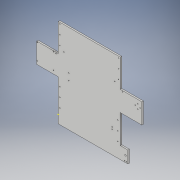
# Autodesk Inventor part: Gen2PlatePart
Saved by Autodesk Inventor 2017 (Build 210142000, 142)
## iProperties
Created: 2017-12-06
Part Number: Gen2PlatePart
Material: Generic
Document SubType Name: Modeling
Designer: User
Density: 1 g/cm^3
Appearance: Default
Author: User
Autodesk Inventor part; units mm, degrees
ref_plane "YZ Plane" through (0, 0, 0) normal (1, 0, 0) x (0, 1, 0)
ref_plane "XZ Plane" through (0, 0, 0) normal (0, 1, 0) x (-1, 0, 0)
ref_plane "XY Plane" through (0, 0, 0) normal (0, 0, 1) x (1, 0, 0)
sketch "Sketch1" plane through (0, 0, 0) normal (0, 0, 1) x (1, 0, 0)
  line L0 (0, 0) -> (254, 0)
  line L1 (254, 0) -> (254, 330.2)
  line L2 (254, 330.2) -> (0, 330.2)
  line L3 (0, 330.2) -> (0, 0)
  dimension "d0" = 254
  dimension "d1" = 330.2
  constraints: 8 end point, 2 parallel, 1 horizontal, 1 perpendicular
  measures "d0" distance of L2.end L1.end
  measures "d1" distance of L1.end L0.end
extrude "Extrusion1" add sketch "Sketch1" along normal blind 6.35
sketch "Sketch2" plane through (0, 0, 6.35) normal (0, 0, 1) x (1, 0, 0)
  point P0 (0, 0)
sketch "Sketch3" plane through (0, 0, 0) normal (-1, 0, 0) x (0, 0, 1)
  line L0 (0, 0) -> (0, 330.2) projected
  line L1 (0, 330.2) -> (-38.1, 330.2)
  line L2 (-38.1, 330.2) -> (38.1, 330.2)
  line L3 (38.1, 330.2) -> (38.1, 266.7)
  line L4 (38.1, 266.7) -> (-38.1, 266.7)
  line L5 (-38.1, 266.7) -> (-38.1, 330.2)
  line L6 (-38.1, 0) -> (38.1, 0)
  line L7 (38.1, 0) -> (38.1, 63.5)
  line L8 (38.1, 63.5) -> (-38.1, 63.5)
  line L9 (-38.1, 63.5) -> (-38.1, 0)
  dimension "d4" = 38.1
  dimension "d5" = 76.2
  dimension "d6" = 63.5
  dimension "d9" = 63.5
  constraints: 18 end point, 4 parallel, 3 horizontal, 2 perpendicular
  measures "d4" distance of L0.end L1.end
  measures "d5" distance of L3.end L4.end
  measures "d6" distance of L2.end L3.end
  measures "d9" distance of L7.end L6.end
extrude "Extrusion2" add sketch "Sketch3" against normal blind 6.35
sketch "Sketch4" plane through (6.35, 0, 0) normal (0, -1, 0) x (1, 0, 0)
  line L0 (0, -38.1) -> (0, 0) projected
  line L1 (247.65, 6.35) -> (0, 6.35) projected
  line L2 (0, 0) -> (38.1, 0)
  line L3 (38.1, 0) -> (38.1, 6.35)
  line L4 (38.1, 6.35) -> (0, 6.35)
  line L5 (0, 6.35) -> (0, 0)
  point P0 (-6.35, 0)
  dimension "d10" = 38.1
  constraints: 8 end point, 2 parallel, 1 horizontal, 1 perpendicular, 1 point on line
  measures "d10" distance of L4.end L3.end
extrude "Extrusion3" cut sketch "Sketch4" against normal blind 38.1
sketch "Sketch5" plane through (6.35, 330.2, 0) normal (0, 1, 0) x (1, 0, 0)
  line L0 (0, 0) -> (-6.35, 0) projected
  line L1 (0, -6.35) -> (38.1, -6.35) projected
  line L2 (0, 0) -> (38.1, 0)
  line L3 (38.1, 0) -> (38.1, -6.35)
  line L4 (38.1, -6.35) -> (0, -6.35)
  line L5 (0, -6.35) -> (0, 0)
  constraints: 8 end point, 2 parallel, 1 horizontal, 1 perpendicular
extrude "Extrusion4" cut sketch "Sketch5" against normal blind 38.1
sketch "Sketch6" plane through (254, 0, 0) normal (1, 0, 0) x (0, 0, -1)
  line L0 (38.1, 0) -> (-38.1, 0) projected
  line L1 (38.1, 63.5) -> (0, 63.5) projected
  line L2 (-38.1, 0) -> (38.1, 0)
  line L3 (38.1, 0) -> (38.1, 63.5)
  line L4 (38.1, 63.5) -> (-38.1, 63.5)
  line L5 (-38.1, 63.5) -> (-38.1, 0)
  line L6 (-38.1, 266.7) -> (-6.35, 266.7) projected
  line L7 (38.1, 330.2) -> (-38.1, 330.2) projected
  line L8 (-38.1, 266.7) -> (38.1, 266.7)
  line L9 (38.1, 266.7) -> (38.1, 330.2)
  line L10 (38.1, 330.2) -> (-38.1, 330.2)
  line L11 (-38.1, 330.2) -> (-38.1, 266.7)
  point P0 (0, 0)
  constraints: 16 end point, 4 parallel, 2 horizontal, 2 perpendicular
extrude "Extrusion5" add sketch "Sketch6" against normal blind 6.35
sketch "Sketch7" plane through (44.45, 330.2, 6.35) normal (0, 1, 0) x (1, 0, 0)
  line L0 (0, 0) -> (203.2, 0) projected
  line L1 (0, 6.35) -> (203.2, 6.35) projected
  line L2 (203.2, 0) -> (165.1, 0)
  line L3 (165.1, 0) -> (165.1, 6.35)
  line L4 (165.1, 6.35) -> (203.2, 6.35)
  line L5 (203.2, 6.35) -> (203.2, 0)
  point P0 (-44.45, 6.35)
  dimension "d17" = 38.1
  constraints: 8 end point, 2 parallel, 1 horizontal, 1 perpendicular, 1 point on line
  measures "d17" distance of L3.end L4.end
extrude "Extrusion6" cut sketch "Sketch7" against normal blind 38.1
sketch "Sketch8" plane through (44.45, 0, 0) normal (0, -1, 0) x (1, 0, 0)
  line L0 (209.55, 0) -> (203.2, 0) projected
  line L1 (0, 6.35) -> (203.2, 6.35) projected
  line L2 (203.2, 0) -> (165.1, 0)
  line L3 (165.1, 0) -> (165.1, 6.35)
  line L4 (165.1, 6.35) -> (203.2, 6.35)
  line L5 (203.2, 6.35) -> (203.2, 0)
  point P0 (-44.45, 0)
  dimension "d20" = 38.1
  constraints: 8 end point, 2 parallel, 1 horizontal, 1 perpendicular, 1 point on line
  measures "d20" distance of L3.end L4.end
extrude "Extrusion7" cut sketch "Sketch8" against normal blind 38.1
sketch "Sketch9" plane through (6.35, 0, 0) normal (1, 0, 0) x (0, 0, -1)
  line L0 (38.1, 0) -> (-38.1, 0) projected
  line L1 (-19.0903, 0) -> (-19.0903, 17.1196)
  line L2 (-19.0903, 0) -> (-1.9707, 0) construction
  line L3 (-38.1, 63.5) -> (-38.1, 0) projected
  line L4 (-38.1, 17.1196) -> (-20.955, 17.1196)
  line L5 (-38.1, 17.1196) -> (-20.955, 17.1196) construction
  circle A0 centre (-20.955, 17.1196) radius 3.4925
  point P0 (0, 0)
  dimension "d23" = 17.1196
  dimension "d24" = 90
  dimension "d25" = 17.145
  dimension "d26" = 0
  dimension "d27" = 6.985
  constraints: 8 end point, 2 equal length, 2 horizontal, 2 perpendicular, 2 point on line, 1 centre point, 1 coincident
  measures "d23" distance of L1.start L1.end
  measures "d24" angle of L2 L1
  measures "d25" distance of L4.start L4.end
  measures "d26" distance between parallel lines of L4 L5
  measures "d27" diameter of A0
extrude "Extrusion8" cut sketch "Sketch9" against normal blind 38.1 contours A0
sketch "Sketch10" plane through (6.35, 0, 0) normal (1, 0, 0) x (0, 0, -1)
  circle A0 centre (-20.955, 17.1196) radius 3.4925 projected
  circle A1 centre (-20.955, 17.1196) radius 8
  circle A2 centre (-20.955, 9.1196) radius 1.5875
  circle A3 centre (-14.0268, 13.1196) radius 1.5875
  circle A4 centre (-20.955, 17.1196) radius 8
  circle A5 centre (-14.0268, 21.1196) radius 1.5875
  circle A6 centre (-20.955, 17.1196) radius 8
  circle A7 centre (-20.955, 25.1196) radius 1.5875
  circle A8 centre (-20.955, 17.1196) radius 8
  circle A9 centre (-27.8832, 21.1196) radius 1.5875
  circle A10 centre (-20.955, 17.1196) radius 8
  circle A11 centre (-27.8832, 13.1196) radius 1.5875
  circle A12 centre (-20.955, 17.1196) radius 8
  point P0 (0, 0)
  point P1 (-28.955, 17.1196)
  point P2 (-24.955, 10.1914)
  point P3 (-16.955, 10.1914)
  point P4 (-12.955, 17.1196)
  point P5 (-16.955, 24.0478)
  point P6 (-24.955, 24.0478)
  dimension "d33" = 3.175
  dimension "d36" = 360
  constraints: 12 centre point, 12 point on circle, 9 coincident, 35 other
  measures "d33" diameter of A2
extrude "Extrusion9" cut sketch "Sketch10" against normal blind 38.1 contours A5 A1 | A1 A5 | A3 A1 | A1 A3 | A7 A1 | A1 A7 | A2 A1 | A1 A2 | A9 A1 | A1 A9 | A11 A1 | A1 A11
sketch "Sketch11" plane through (247.65, 0, 0) normal (-1, 0, 0) x (0, 0, 1)
  line L0 (38.1, 0) -> (38.1, 63.5) projected
  line L1 (38.1, 17.1196) -> (70.485, 17.1196) construction
  circle A0 centre (20.955, 17.1196) radius 3.4925
  circle A1 centre (20.955, 17.1196) radius 8.001
  line L2 (20.955, 17.1196) -> (31.4906, 17.1196)
  circle A2 centre (28.956, 17.1196) radius 1.5875
  circle A3 centre (24.9555, 24.0487) radius 1.5875
  circle A4 centre (20.955, 17.1196) radius 8.001
  circle A5 centre (16.9545, 24.0487) radius 1.5875
  circle A6 centre (20.955, 17.1196) radius 8.001
  circle A7 centre (12.954, 17.1196) radius 1.5875
  circle A8 centre (20.955, 17.1196) radius 8.001
  circle A9 centre (16.9545, 10.1905) radius 1.5875
  circle A10 centre (20.955, 17.1196) radius 8.001
  circle A11 centre (24.9555, 10.1905) radius 1.5875
  circle A12 centre (20.955, 17.1196) radius 8.001
  point P0 (0, 0)
  point P1 (20.955, 9.1186)
  point P2 (27.8841, 13.1191)
  point P3 (27.8841, 21.1201)
  point P4 (20.955, 25.1206)
  point P5 (14.0259, 21.1201)
  point P6 (14.0259, 13.1191)
  dimension "d44" = 16.002
  dimension "d41" = 17.145
  dimension "d43" = 6.985
  dimension "d81" = 3.175
  dimension "d84" = 360
  constraints: 7 centre point, 4 end point, 3 coincident, 2 point on line, 2 vertical alignment, 1 horizontal, 47 other
  measures "d41" distance of L1.start point (20.955, 17.12)
  measures "d43" diameter of A0
  measures "d81" diameter of A2
extrude "Extrusion10" cut sketch "Sketch11" against normal blind 25.4 contours A0 | L2 A2 A1 | L2 A2 A1 | A1 A2 L2 | A1 A2 L2 | A3 A1 | A1 A3 | A11 A1 | A1 A11 | A5 A1 | A1 A5 | A9 A1 | A1 A9 | A7 A1 | A1 A7
sketch "Sketch12" plane through (254, 63.5, 0) normal (1, 0, 0) x (0, 0, -1)
  line L0 (-38.1, 266.7) -> (-38.1, 203.2) projected
  line L1 (-38.1, 234.95) -> (-20.955, 234.95)
  line L2 (0, 228.6) -> (0, 266.7) projected
  line L3 (38.1, 266.7) -> (-38.1, 266.7) projected
  line L4 (-20.955, 266.7) -> (-20.955, 249.5804)
  line L5 (-20.955, 266.7) -> (-3.8354, 266.7) construction
  circle A0 centre (-20.955, 249.5804) radius 3.4925
  circle A1 centre (-20.955, 249.5804) radius 8.001
  line L6 (-20.955, 234.95) -> (-20.955, 230.7922)
  line L7 (-20.955, 249.5804) -> (-30.6683, 249.5804)
  line L8 (-6.35, 266.7) -> (-6.35, 228.6) projected
  circle A2 centre (-20.955, 257.5814) radius 1.5875
  circle A3 centre (-27.8841, 253.5809) radius 1.5875
  circle A4 centre (-20.955, 249.5804) radius 8.001
  circle A5 centre (-27.8841, 245.5799) radius 1.5875
  circle A6 centre (-20.955, 249.5804) radius 8.001
  circle A7 centre (-20.955, 241.5794) radius 1.5875
  circle A8 centre (-20.955, 249.5804) radius 8.001
  circle A9 centre (-14.0259, 245.5799) radius 1.5875
  circle A10 centre (-20.955, 249.5804) radius 8.001
  circle A11 centre (-14.0259, 253.5809) radius 1.5875
  circle A12 centre (-20.955, 249.5804) radius 8.001
  point P0 (0, -63.5)
  dimension "d56" = 16.002
  dimension "d52" = 17.145
  dimension "d53" = 17.1196
  dimension "d54" = 90
  dimension "d55" = 6.985
  dimension "d80" = 0
  dimension "d104" = 3.175
  dimension "d107" = 360
  constraints: 10 end point, 8 coincident, 7 centre point, 4 perpendicular, 2 point on line, 2 vertical alignment, 1 horizontal, 1 midpoint, 1 vertical, 47 other
  measures "d52" distance of L1.start L1.end
  measures "d53" distance of L4.start L4.end
  measures "d54" angle of L4 L5
  measures "d55" diameter of A0
  measures "d80" distance from line of L4.end L6
  measures "d104" diameter of A2
extrude "Extrusion11" cut sketch "Sketch12" against normal blind 25.4 contours A2 A1 L4 | L4 A1 A2 | A1 A2 L4 | L4 A2 A1 | A3 A1 | A1 A3 | A0 L7 L4 | L4 L7 A0 | A11 A1 | A1 A11 | A5 A1 | A1 A5 | A9 A1 | A1 A9 | A7 A1 | A1 A7
sketch "Sketch13" plane through (0, 63.5, 0) normal (-1, 0, 0) x (0, 0, 1)
  line L0 (-38.1, 266.7) -> (38.1, 266.7) projected
  line L1 (23.9735, 266.7) -> (41.0931, 266.7) construction
  line L2 (38.1, 249.5804) -> (20.955, 249.5804)
  line L3 (38.1, 249.5804) -> (55.245, 249.5804) construction
  circle A0 centre (20.955, -46.3804) radius 3.4925 projected
  line L4 (38.1, -63.5) -> (38.1, 0) projected
  circle A1 centre (20.955, 249.5804) radius 3.4925
  circle A2 centre (20.955, 249.5804) radius 8.001
  circle A3 centre (28.956, 249.5804) radius 1.5875
  circle A4 centre (24.9555, 256.5095) radius 1.5875
  circle A5 centre (20.955, 249.5804) radius 8.001
  circle A6 centre (16.9545, 256.5095) radius 1.5875
  circle A7 centre (20.955, 249.5804) radius 8.001
  circle A8 centre (12.954, 249.5804) radius 1.5875
  circle A9 centre (20.955, 249.5804) radius 8.001
  circle A10 centre (16.9545, 242.6513) radius 1.5875
  circle A11 centre (20.955, 249.5804) radius 8.001
  circle A12 centre (24.9555, 242.6513) radius 1.5875
  circle A13 centre (20.955, 249.5804) radius 8.001
  line L5 (38.1, 203.2) -> (6.35, 203.2) projected
  point P0 (0, -63.5)
  point P1 (20.9804, 257.5814)
  point P2 (14.0387, 253.6029)
  point P3 (14.0133, 245.6019)
  point P4 (20.9296, 241.5794)
  point P5 (27.8713, 245.5579)
  point P6 (27.8967, 253.5589)
  dimension "d67" = 17.145
  dimension "d68" = 180
  dimension "d69" = 17.145
  dimension "d70" = 6.985
  dimension "d71" = 6.985
  dimension "d72" = 16.002
  dimension "d92" = 3.175
  dimension "d95" = 360
  dimension "d134" = 46.3804
  constraints: 13 centre point, 12 point on circle, 6 end point, 3 horizontal, 2 coincident, 2 point on line, 1 collinear, 31 other
  measures "d67" distance of L2.start L2.end
  measures "d68" angle of L2 L3
  measures "d69" distance from line of A0.centre L4
  measures "d70" diameter of A0
  measures "d71" diameter of A1
  measures "d72" diameter of A2
  measures "d92" diameter of A3
  measures "d134" distance from line of L5 L2.end
extrude "Extrusion12" cut sketch "Sketch13" against normal blind 25.4 contours A3 A2 L2 | L2 A2 A3 | A2 A3 L2 | L2 A3 A2 | A4 A2 | A2 A4 | A12 A2 | A2 A12 | A6 A2 | A2 A6 | A10 A2 | A2 A10 | A8 A2 | A2 A8 | A1
sketch "Sketch14" plane through (254, 63.5, 0) normal (1, 0, 0) x (0, 0, -1)
  line L0 (0, -63.5) -> (0, 50.8)
  line L1 (0, 203.2) -> (0, 0) projected
  line L2 (38.1, 266.7) -> (-38.1, 266.7) projected
  line L3 (0, 266.7) -> (0, 165.1)
  line L4 (-6.35, 203.2) -> (-6.35, 0) projected
  line L5 (0, 50.8) -> (-6.35, 50.8)
  line L6 (-6.35, 241.3) -> (0, 241.3)
  line L7 (0, 266.7) -> (-6.35, 266.7) projected
  line L8 (0, 266.7) -> (0, 152.4)
  line L9 (0, 0) -> (0, 203.2) projected
  line L10 (-6.35, 0) -> (-6.35, 203.2) projected
  line L11 (0, 50.8) -> (-6.35, 50.8)
  line L12 (-6.35, 152.4) -> (0, 152.4)
  line L13 (0, 152.4) -> (0, 69.85)
  line L14 (0, 69.85) -> (-6.35, 69.85)
  line L15 (-6.35, 69.85) -> (-6.35, 152.4)
  dimension "d109" = 114.3
  dimension "d137" = 114.3
  dimension "d305" = 82.55
  constraints: 20 end point, 5 point on line, 2 horizontal, 2 parallel, 1 collinear, 1 midpoint, 1 perpendicular
  measures "d109" distance of L0.start L0.end
  measures "d137" distance of L3.start L8.end
  measures "d305" distance of L12.end L13.end
sketch "Sketch15" plane through (0, 63.5, 0) normal (-1, 0, 0) x (0, 0, 1)
  line L0 (0, -63.5) -> (0, 38.1)
  line L1 (0, 0) -> (0, -25.4) projected
  line L2 (-38.1, 266.7) -> (38.1, 266.7) projected
  line L3 (0, 266.7) -> (0, 165.1)
  line L4 (0, 266.7) -> (0, 228.6) projected
  line L5 (0, 165.1) -> (6.35, 165.1)
  line L6 (6.35, 38.1) -> (0, 38.1)
  line L7 (0, 165.1) -> (0, 69.85)
  line L8 (0, 69.85) -> (6.35, 69.85)
  line L9 (6.35, 165.1) -> (6.35, 69.85)
  line L10 (6.35, 203.2) -> (6.35, 0) projected
  dimension "d113" = 101.6
  dimension "d114" = 101.6
  dimension "d306" = 95.25
  constraints: 14 end point, 3 collinear, 1 horizontal, 1 midpoint, 1 parallel
  measures "d113" distance of L0.start L0.end
  measures "d114" distance of L3.start L3.end
  measures "d306" distance of L3.end L7.end
extrude "Extrusion14" add sketch "Sketch15" along normal blind 88.9
thicken "Thicken1" operation add thickness 22.225 both sides no extend neighbours yes toward (0, 0, 1) faces at (251.8833, 287.8667, -38.1)
thicken "Thicken2" operation add thickness 22.225 both sides no extend neighbours yes toward (0, 0, 1) faces at (2.1167, 287.8667, -38.1)
thicken "Thicken3" operation add thickness 22.225 both sides no extend neighbours yes toward (0, 0, 1) faces at (2.1167, 42.3333, -38.1)
thicken "Thicken4" operation add thickness 22.225 both sides no extend neighbours yes toward (0, 0, 1) faces at (251.8833, 21.1667, -38.1)
extrude "Extrusion15" add sketch "Sketch14" along normal blind 88.9 contours L1 L14 L4 L12
thicken "Thicken10" operation add thickness 12.7 both sides no extend neighbours yes toward (0, -1, 0) faces at (-29.6333, 228.6, 4.2333)
thicken "Thicken12" operation add thickness 15.875 both sides no extend neighbours yes toward (0, 0, 1) faces at (249.7667, 309.0333, -15.875)
thicken "Thicken13" operation add thickness 15.875 both sides no extend neighbours yes toward (0, 0, 1) faces at (4.2333, 287.8667, -15.875)
thicken "Thicken14" operation add thickness 15.875 both sides no extend neighbours yes toward (0, 0, 1) faces at (251.8833, 21.1667, -15.875)
thicken "Thicken15" operation add thickness 15.875 both sides no extend neighbours yes toward (0, 0, 1) faces at (2.1167, 42.3333, -15.875)
thicken "Thicken16" operation add thickness 38.1 both sides no extend neighbours yes toward (-1, 0, 0) faces at (44.45, 25.4, 2.1167)
thicken "Thicken17" operation add thickness 38.1 both sides no extend neighbours yes toward (1, 0, 0) faces at (209.55, 25.4, 2.1167)
thicken "Thicken18" operation add thickness 38.1 both sides no extend neighbours yes toward (1, 0, 0) faces at (209.55, 317.5, 2.1167)
thicken "Thicken19" operation add thickness 38.1 both sides no extend neighbours yes toward (-1, 0, 0) faces at (44.45, 317.5, 2.1167)
thicken "Thicken20" operation add thickness 34.925 both sides no extend neighbours yes toward (0, -1, 0) faces at (86.7833, 0, 2.1167)
thicken "Thicken21" operation add thickness 12.7 both sides no extend neighbours yes toward (0, -1, 0) faces at (167.2167, -34.925, 2.1167)
thicken "Thicken22" operation add thickness 31.75 both sides no extend neighbours yes toward (0, 0, -1) faces at (2.1167, 309.0333, 38.1)
thicken "Thicken23" operation add thickness 31.75 both sides no extend neighbours yes toward (0, 0, -1) faces at (249.7667, 309.0333, 38.1)
thicken "Thicken24" operation add thickness 31.75 both sides no extend neighbours yes toward (0, 0, -1) faces at (4.2333, 26.4583, 38.1)
thicken "Thicken25" operation add thickness 31.75 both sides no extend neighbours yes toward (0, 0, -1) faces at (249.7667, -10.5833, 38.1)
sketch "Sketch20" plane through (0, 330.2, 6.35) normal (0, 0, 1) x (1, 0, 0)
  line L0 (0, -114.3) -> (0, 0) projected
  line L1 (0, 0) -> (12.7, 0)
  line L2 (12.7, 0) -> (12.7, -88.9)
  line L3 (12.7, -88.9) -> (0, -88.9)
  line L4 (0, -88.9) -> (0, 0)
  line L5 (254, -114.3) -> (254, 0) projected
  line L6 (254, 0) -> (241.3, 0)
  line L7 (241.3, 0) -> (241.3, -88.9)
  line L8 (241.3, -88.9) -> (254, -88.9)
  line L9 (254, -88.9) -> (254, 0)
  line L10 (254, -377.825) -> (254, 0) projected
  line L11 (254, -222.25) -> (233.7253, -222.25)
  line L12 (233.7253, -222.25) -> (233.7253, -311.15)
  line L13 (233.7253, -311.15) -> (254, -311.15)
  line L14 (254, -311.15) -> (254, -222.25)
  line L15 (0, -196.85) -> (0, -377.825) projected
  line L16 (0, -222.25) -> (12.7, -222.25)
  line L17 (12.7, -222.25) -> (12.7, -311.15)
  line L18 (12.7, -311.15) -> (0, -311.15)
  line L19 (0, -311.15) -> (0, -222.25)
  line L20 (6.35, -311.15) -> (6.35, -304.8)
  line L21 (0, -266.7) -> (12.7, -266.7)
  line L22 (6.35, -222.25) -> (6.35, -228.6)
  line L23 (233.7253, -266.7) -> (254, -266.7)
  line L24 (243.8627, -311.15) -> (243.8627, -304.8)
  line L25 (243.8627, -222.25) -> (243.8627, -228.6)
  line L26 (247.65, 0) -> (247.65, -6.35)
  line L27 (241.3, -44.45) -> (254, -44.45)
  line L28 (247.65, -88.9) -> (247.65, -82.55)
  line L29 (6.35, 0) -> (6.35, -6.35)
  line L30 (0, -44.45) -> (12.7, -44.45)
  line L31 (6.35, -88.9) -> (6.35, -82.55)
  line L32 (254, -215.9) -> (342.9, -215.9) projected
  line L33 (243.8627, -228.6) -> (6.35, -228.6)
  point P0 (0, -330.2)
  point P1 (0, -228.6)
  point P2 (6.35, -266.7)
  point P3 (243.8627, -266.7)
  point P4 (247.65, -44.45)
  point P5 (6.35, -44.45)
  dimension "d200" = 12.7
  dimension "d201" = 88.9
  dimension "d202" = 12.7
  dimension "d203" = 88.9
  dimension "d204" = 88.9
  dimension "d208" = 6.35
  dimension "d209" = 6.35
  dimension "d210" = 6.35
  dimension "d211" = 6.35
  dimension "d212" = 6.35
  dimension "d213" = 6.35
  dimension "d214" = 0
  dimension "d216" = 6.35
  dimension "d217" = 0
  dimension "d311" = 38.1
  dimension "d312" = 38.1
  dimension "d313" = 6.35
  dimension "d314" = 6.35
  dimension "d315" = 38.1
  dimension "d316" = 38.1
  dimension "d317" = 38.1
  dimension "d318" = 0
  constraints: 58 end point, 20 midpoint, 8 coincident, 8 parallel, 8 vertical, 5 horizontal, 4 perpendicular
  measures "d200" distance of L2.end L3.end
  measures "d201" distance of L1.end L2.end
  measures "d202" distance of L8.end L7.end
  measures "d203" distance of L7.end L6.end
  measures "d204" distance of L12.end L11.end
  measures "d208" distance of L24.start L24.end
  measures "d209" distance of L25.start L25.end
  measures "d210" distance of L26.start L26.end
  measures "d211" distance of L28.start L28.end
  measures "d212" distance of L29.start L29.end
  measures "d213" distance of L31.start L31.end
  measures "d214" distance between parallel lines of L15 L19
  measures "d216" distance between parallel lines of L32 L11
  measures "d217" distance between parallel lines of L10 L14
  measures "d311" distance of point (6.35, -266.7) point (6.35, -228.6)
  measures "d312" distance of point (6.35, -266.7) point (6.35, -304.8)
  measures "d313" distance of point (6.35, -228.6) L22.start
  measures "d314" distance of L20.start point (6.35, -304.8)
  measures "d315" distance of L33.start point (243.863, -266.7)
  measures "d316" distance of point (243.863, -304.8) point (243.863, -266.7)
  measures "d317" distance of point (6.35, -6.35) point (6.35, -44.45)
  measures "d318" distance of point (6.35, -228.6) L33.end
hole "Hole3" at (6.35, 323.85, 6.35) at (6.35, 285.75, 6.35) at (6.35, 247.65, 6.35) at (6.35, 101.6, 6.35) at (6.35, 63.5, 6.35) at (6.35, 25.4, 6.35) at (247.65, 285.75, 6.35) at (247.65, 323.85, 6.35) at (247.65, 247.65, 6.35) at (243.8627, 101.6, 6.35) at (243.8627, 63.5, 6.35) at (243.8627, 25.4, 6.35) direction (0, 0, -1) diameter 3.302 depth 25.4 tip angle 118
sketch "Sketch22" plane through (0, 330.2, 6.35) normal (0, 0, 1) x (1, 0, 0)
  line L0 (254, -114.3) -> (342.9, -114.3) projected
  line L1 (342.9, -114.3) -> (342.9, -215.9) projected
  circle A0 centre (335.915, -139.7) radius 1.778
  circle A1 centre (316.357, -139.7) radius 1.778
  circle A2 centre (325.882, -130.175) radius 1.778
  circle A3 centre (325.882, -149.225) radius 1.778
  point P0 (0, -330.2)
  dimension "d236" = 25.4
  dimension "d237" = 6.985
  dimension "d238" = 3.556
  dimension "d239" = 26.543
  dimension "d240" = 3.556
  dimension "d241" = 9.525
  dimension "d242" = 9.525
  dimension "d243" = 3.556
  dimension "d244" = 9.525
  dimension "d245" = 9.525
  dimension "d246" = 3.556
  constraints: 4 centre point, 4 coincident
  measures "d236" distance from line of L0 point (335.915, -139.7)
  measures "d237" distance from line of point (335.915, -139.7) L1
  measures "d238" diameter of A0
  measures "d239" distance from line of L1 point (316.357, -139.7)
  measures "d240" diameter of A1
  measures "d241" horizontal distance of point (325.882, -130.175) point (316.357, -139.7)
  measures "d242" horizontal distance of point (316.357, -139.7) point (325.882, -130.175)
  measures "d243" diameter of A2
  measures "d244" horizontal distance of point (325.882, -149.225) A1.centre
  measures "d245" horizontal distance of A1.centre point (325.882, -149.225)
  measures "d246" diameter of A3
extrude "Extrusion17" cut sketch "Sketch22" against normal blind 25.4
sketch "Sketch23" plane through (0, 330.2, 6.35) normal (0, 0, 1) x (1, 0, 0)
  circle A0 centre (325.882, -130.175) radius 1.778 projected
  circle A1 centre (335.915, -139.7) radius 1.778 projected
  circle A2 centre (316.357, -139.7) radius 1.778 projected
  circle A3 centre (325.882, -149.225) radius 1.778 projected
  circle A4 centre (243.8627, -266.7) radius 1.651 projected
  circle A5 centre (247.65, -82.55) radius 1.651 projected
  circle A6 centre (247.65, -44.45) radius 1.651 projected
  circle A7 centre (6.35, -266.7) radius 1.651 projected
  circle A8 centre (6.35, -82.55) radius 1.651 projected
  circle A9 centre (6.35, -6.35) radius 1.651 projected
  circle A10 centre (6.35, -44.45) radius 1.651 projected
  circle A11 centre (6.35, -228.6) radius 1.651 projected
  circle A12 centre (6.35, -304.8) radius 1.651 projected
  circle A13 centre (247.65, -6.35) radius 1.651 projected
  circle A14 centre (243.8627, -228.6) radius 1.651 projected
  circle A15 centre (243.8627, -304.8) radius 1.651 projected
  line L0 (254, 0) -> (254, -114.3) projected
  line L1 (254, -114.3) -> (342.9, -114.3) projected
  line L2 (0, 0) -> (254, 0) projected
  line L3 (0, 0) -> (0, -114.3) projected
  line L4 (0, -114.3) -> (-88.9, -114.3) projected
  line L5 (254, -377.825) -> (0, -377.825) projected
  line L6 (254, -196.85) -> (342.9, -196.85) projected
  line L7 (342.9, -114.3) -> (342.9, -196.85) projected
  line L8 (-88.9, -196.85) -> (-88.9, -114.3) projected
  line L9 (0, -196.85) -> (-88.9, -196.85) projected
  line L10 (0, -377.825) -> (0, -196.85) projected
  line L11 (254, -377.825) -> (254, -196.85) projected
  point P0 (0, -330.2)
  point P1 (263.1059, -119.0625)
  point P2 (231.3559, -97.4725)
  point P3 (22.6441, -97.4725)
  point P4 (-9.1059, -119.0625)
  dimension "d250" = 4.7625
  dimension "d252" = 16.8275
  dimension "d253" = 22.6441
  measures "d250" distance from line of L1 point (263.106, -119.062)
  measures "d252" distance from line of L1 point (231.356, -97.472)
  measures "d253" distance from line of L3 point (22.644, -97.472)
hole "Hole4" at (-9.1059, 211.1375, 6.35) at (22.6441, 232.7275, 6.35) at (231.3559, 232.7275, 6.35) at (263.1059, 211.1375, 6.35) direction (0, 0, -1) diameter 3.556 end through all
sketch "Sketch24" plane through (254, -47.625, 0) normal (1, 0, 0) x (0, 0, -1)
  line L0 (0, 0) -> (0, 377.825) projected
  line L1 (-6.35, 0) -> (-6.35, 180.975) projected
  line L2 (0, 0) -> (-6.35, 0)
  line L3 (-6.35, 0) -> (-6.35, 44.45)
  line L4 (-6.35, 44.45) -> (0, 44.45)
  line L5 (0, 44.45) -> (0, 0)
  point P0 (0, 47.625)
  point P1 (0, 161.925)
  point P2 (-6.35, 161.925)
  dimension "d262" = 44.45
  constraints: 8 end point, 2 parallel, 1 horizontal, 1 perpendicular, 1 point on line
  measures "d262" distance of L2.end L3.end
extrude "Extrusion18" add sketch "Sketch24" along normal blind 31.75
sketch "Sketch26" plane through (0, 330.2, 6.35) normal (0, 0, 1) x (1, 0, 0)
  line L0 (285.75, -377.825) -> (285.75, -333.375) projected
  line L1 (285.75, -358.648) -> (279.4, -358.648)
  line L2 (285.75, -358.648) -> (292.1, -358.648) construction
  line L3 (285.75, -377.825) -> (0, -377.825) projected
  point P0 (0, -330.2)
  point P1 (272.1, -358.648)
  dimension "d270" = 6.35
  dimension "d271" = 180
  dimension "d302" = 19.177
  dimension "d303" = 19.177
  constraints: 4 end point, 1 coincident, 1 collinear, 1 horizontal, 1 perpendicular, 1 point on line
  measures "d270" distance of L1.start L1.end
  measures "d271" angle of L1 L2
  measures "d302" distance from line of L3 L1.end
  measures "d303" distance from line of L3 point (272.1, -358.648)
hole "Hole5" at (272.1, -28.448, 6.35) at (279.4, -28.448, 6.35) direction (0, 0, -1) diameter 3.556 depth 6.35 tip angle 118
sketch "Sketch27" plane through (0, 330.2, 6.35) normal (0, 0, 1) x (1, 0, 0)
  point P0 (0, -330.2)
thicken "Thicken26" operation add thickness 5.08 both sides no extend neighbours yes toward (0, -1, 0) faces at (190.5, -47.625, 2.1167)
sketch "Sketch29" plane through (0, 330.2, 6.35) normal (0, 0, 1) x (1, 0, 0)
  circle A0 centre (272.1, -358.648) radius 1.778 projected
  circle A1 centre (279.4, -358.648) radius 1.778 projected
  circle A2 centre (231.3559, -97.4725) radius 1.778 projected
  circle A3 centre (-9.1059, -119.0625) radius 1.778 projected
  circle A4 centre (22.6441, -97.4725) radius 1.778 projected
  circle A5 centre (263.1059, -119.0625) radius 1.778 projected
  circle A6 centre (325.882, -130.175) radius 1.778 projected
  circle A7 centre (335.915, -139.7) radius 1.778 projected
  circle A8 centre (316.357, -139.7) radius 1.778 projected
  circle A9 centre (325.882, -149.225) radius 1.778 projected
  circle A10 centre (243.8627, -266.7) radius 1.651 projected
  circle A11 centre (247.65, -82.55) radius 1.651 projected
  circle A12 centre (247.65, -44.45) radius 1.651 projected
  circle A13 centre (6.35, -266.7) radius 1.651 projected
  circle A14 centre (6.35, -82.55) radius 1.651 projected
  circle A15 centre (6.35, -6.35) radius 1.651 projected
  circle A16 centre (6.35, -44.45) radius 1.651 projected
  circle A17 centre (6.35, -228.6) radius 1.651 projected
  circle A18 centre (6.35, -304.8) radius 1.651 projected
  circle A19 centre (247.65, -6.35) radius 1.651 projected
  circle A20 centre (243.8627, -228.6) radius 1.651 projected
  circle A21 centre (243.8627, -304.8) radius 1.651 projected
  line L0 (254, -333.375) -> (254, -196.85) projected
  line L1 (254, -114.3) -> (342.9, -114.3) projected
  line L2 (254, 0) -> (254, -114.3) projected
  line L3 (0, 0) -> (254, 0) projected
  line L4 (0, 0) -> (0, -114.3) projected
  line L5 (0, -114.3) -> (-88.9, -114.3) projected
  line L6 (285.75, -382.905) -> (0, -382.905) projected
  line L7 (285.75, -333.375) -> (285.75, -382.905) projected
  line L8 (254, -333.375) -> (285.75, -333.375) projected
  line L9 (254, -196.85) -> (342.9, -196.85) projected
  line L10 (342.9, -114.3) -> (342.9, -196.85) projected
  line L11 (-88.9, -196.85) -> (-88.9, -114.3) projected
  line L12 (0, -196.85) -> (-88.9, -196.85) projected
  line L13 (0, -382.905) -> (0, -196.85) projected
  point P0 (0, -330.2)
  point P1 (275.75, -337.98)
  dimension "d293" = 10
  dimension "d294" = 44.925
  measures "d293" distance from line of point (275.75, -337.98) L7
  measures "d294" distance from line of L6 point (275.75, -337.98)
hole "Hole7" at (275.75, -7.78, 6.35) direction (0, 0, -1) diameter 6.7564 end through all
thicken "Thicken27" operation add thickness 19.05 both sides no extend neighbours yes toward (0, 1, 0) faces at (95.25, -52.705, 4.2333)
thicken "Thicken28" operation add thickness 19.05 both sides no extend neighbours yes toward (0, 1, 0) faces at (264.5833, -3.175, 4.2333)
sketch "Sketch30" plane through (0, 330.2, 6.35) normal (0, 0, 1) x (1, 0, 0)
  circle A0 centre (275.75, -337.98) radius 3.3782 projected
  circle A1 centre (272.1, -358.648) radius 1.778 projected
  circle A2 centre (279.4, -358.648) radius 1.778 projected
  circle A3 centre (231.3559, -97.4725) radius 1.778 projected
  circle A4 centre (-9.1059, -119.0625) radius 1.778 projected
  circle A5 centre (22.6441, -97.4725) radius 1.778 projected
  circle A6 centre (263.1059, -119.0625) radius 1.778 projected
  circle A7 centre (325.882, -130.175) radius 1.778 projected
  circle A8 centre (335.915, -139.7) radius 1.778 projected
  circle A9 centre (316.357, -139.7) radius 1.778 projected
  circle A10 centre (325.882, -149.225) radius 1.778 projected
  circle A11 centre (243.8627, -266.7) radius 1.651 projected
  circle A12 centre (247.65, -82.55) radius 1.651 projected
  circle A13 centre (247.65, -44.45) radius 1.651 projected
  circle A14 centre (6.35, -266.7) radius 1.651 projected
  circle A15 centre (6.35, -82.55) radius 1.651 projected
  circle A16 centre (6.35, -6.35) radius 1.651 projected
  circle A17 centre (6.35, -44.45) radius 1.651 projected
  circle A18 centre (6.35, -228.6) radius 1.651 projected
  circle A19 centre (6.35, -304.8) radius 1.651 projected
  circle A20 centre (247.65, -6.35) radius 1.651 projected
  circle A21 centre (243.8627, -228.6) radius 1.651 projected
  circle A22 centre (243.8627, -304.8) radius 1.651 projected
  line L0 (254, -314.325) -> (254, -196.85) projected
  line L1 (254, -196.85) -> (342.9, -196.85) projected
  line L2 (342.9, -114.3) -> (342.9, -196.85) projected
  line L3 (254, -114.3) -> (342.9, -114.3) projected
  line L4 (254, 0) -> (254, -114.3) projected
  line L5 (0, 0) -> (254, 0) projected
  line L6 (0, 0) -> (0, -114.3) projected
  line L7 (0, -114.3) -> (-88.9, -114.3) projected
  line L8 (-88.9, -196.85) -> (-88.9, -114.3) projected
  line L9 (0, -196.85) -> (-88.9, -196.85) projected
  line L10 (0, -363.855) -> (0, -196.85) projected
  line L11 (285.75, -363.855) -> (0, -363.855) projected
  line L12 (285.75, -314.325) -> (285.75, -363.855) projected
  line L13 (254, -314.325) -> (285.75, -314.325) projected
  point P0 (0, -330.2)
  point P1 (221.107, -272.9738)
  point P2 (221.107, -264.0838)
  dimension "d319" = 90.8812
  dimension "d320" = 8.89
  dimension "d321" = 32.893
  dimension "d322" = 32.893
  measures "d319" distance from line of L11 point (221.107, -272.974)
  measures "d320" distance of point (221.107, -264.084) point (221.107, -272.974)
  measures "d321" distance from line of L0 point (221.107, -264.084)
  measures "d322" distance from line of L0 point (221.107, -272.974)
hole "Hole8" at (221.107, 66.1162, 6.35) at (221.107, 57.2262, 6.35) direction (0, 0, -1) diameter 3.556 depth 25.4 tip angle 118
sketch "Sketch31" plane through (0, 330.2, 6.35) normal (0, 0, 1) x (1, 0, 0)
  circle A0 centre (221.107, -264.0838) radius 1.778 projected
  circle A1 centre (221.107, -272.9738) radius 1.778 projected
  circle A2 centre (275.75, -337.98) radius 3.3782 projected
  circle A3 centre (272.1, -358.648) radius 1.778 projected
  circle A4 centre (279.4, -358.648) radius 1.778 projected
  circle A5 centre (231.3559, -97.4725) radius 1.778 projected
  circle A6 centre (-9.1059, -119.0625) radius 1.778 projected
  circle A7 centre (22.6441, -97.4725) radius 1.778 projected
  circle A8 centre (263.1059, -119.0625) radius 1.778 projected
  circle A9 centre (325.882, -130.175) radius 1.778 projected
  circle A10 centre (335.915, -139.7) radius 1.778 projected
  circle A11 centre (316.357, -139.7) radius 1.778 projected
  circle A12 centre (325.882, -149.225) radius 1.778 projected
  circle A13 centre (243.8627, -266.7) radius 1.651 projected
  circle A14 centre (247.65, -82.55) radius 1.651 projected
  circle A15 centre (247.65, -44.45) radius 1.651 projected
  circle A16 centre (6.35, -266.7) radius 1.651 projected
  circle A17 centre (6.35, -82.55) radius 1.651 projected
  circle A18 centre (6.35, -6.35) radius 1.651 projected
  circle A19 centre (6.35, -44.45) radius 1.651 projected
  circle A20 centre (6.35, -228.6) radius 1.651 projected
  circle A21 centre (6.35, -304.8) radius 1.651 projected
  circle A22 centre (247.65, -6.35) radius 1.651 projected
  circle A23 centre (243.8627, -228.6) radius 1.651 projected
  circle A24 centre (243.8627, -304.8) radius 1.651 projected
  line L0 (254, -314.325) -> (254, -196.85) projected
  line L1 (254, -196.85) -> (342.9, -196.85) projected
  line L2 (342.9, -114.3) -> (342.9, -196.85) projected
  line L3 (254, -114.3) -> (342.9, -114.3) projected
  line L4 (254, 0) -> (254, -114.3) projected
  line L5 (0, 0) -> (254, 0) projected
  line L6 (0, 0) -> (0, -114.3) projected
  line L7 (0, -114.3) -> (-88.9, -114.3) projected
  line L8 (-88.9, -196.85) -> (-88.9, -114.3) projected
  line L9 (0, -196.85) -> (-88.9, -196.85) projected
  line L10 (0, -363.855) -> (0, -196.85) projected
  line L11 (285.75, -363.855) -> (0, -363.855) projected
  line L12 (285.75, -314.325) -> (285.75, -363.855) projected
  line L13 (254, -314.325) -> (285.75, -314.325) projected
  point P0 (0, -330.2)
  point P1 (-85.725, -117.475)
  point P2 (-19.685, -117.475)
  point P3 (-19.685, -183.515)
  point P4 (-85.725, -183.515)
  dimension "d330" = 3.175
  dimension "d331" = 3.175
  dimension "d332" = 3.175
  dimension "d333" = 66.04
  dimension "d334" = 13.335
  dimension "d335" = 13.335
  dimension "d336" = 3.175
  dimension "d337" = 66.04
  measures "d330" distance from line of L7 point (-85.725, -117.475)
  measures "d331" distance from line of L8 point (-85.725, -117.475)
  measures "d332" distance from line of L7 point (-19.685, -117.475)
  measures "d333" distance of point (-19.685, -117.475) point (-85.725, -117.475)
  measures "d334" distance from line of L9 point (-19.685, -183.515)
  measures "d335" distance from line of L9 point (-85.725, -183.515)
  measures "d336" distance from line of L8 point (-85.725, -183.515)
  measures "d337" distance of point (-19.685, -183.515) point (-85.725, -183.515)
hole "Hole9" at (-19.685, 212.725, 6.35) at (-85.725, 212.725, 6.35) at (-19.685, 146.685, 6.35) at (-85.725, 146.685, 6.35) direction (0, 0, -1) diameter 3.556 depth 25.4 tip angle 118
sketch "Sketch32" plane through (0, 330.2, 6.35) normal (0, 0, 1) x (1, 0, 0)
  circle A0 centre (-19.685, -183.515) radius 1.778 projected
  circle A1 centre (-19.685, -117.475) radius 1.778 projected
  circle A2 centre (-85.725, -117.475) radius 1.778 projected
  circle A3 centre (-85.725, -183.515) radius 1.778 projected
  circle A4 centre (221.107, -264.0838) radius 1.778 projected
  circle A5 centre (221.107, -272.9738) radius 1.778 projected
  circle A6 centre (275.75, -337.98) radius 3.3782 projected
  circle A7 centre (272.1, -358.648) radius 1.778 projected
  circle A8 centre (279.4, -358.648) radius 1.778 projected
  circle A9 centre (231.3559, -97.4725) radius 1.778 projected
  circle A10 centre (-9.1059, -119.0625) radius 1.778 projected
  circle A11 centre (22.6441, -97.4725) radius 1.778 projected
  circle A12 centre (263.1059, -119.0625) radius 1.778 projected
  circle A13 centre (325.882, -130.175) radius 1.778 projected
  circle A14 centre (335.915, -139.7) radius 1.778 projected
  circle A15 centre (316.357, -139.7) radius 1.778 projected
  circle A16 centre (325.882, -149.225) radius 1.778 projected
  circle A17 centre (243.8627, -266.7) radius 1.651 projected
  circle A18 centre (247.65, -82.55) radius 1.651 projected
  circle A19 centre (247.65, -44.45) radius 1.651 projected
  circle A20 centre (6.35, -266.7) radius 1.651 projected
  circle A21 centre (6.35, -82.55) radius 1.651 projected
  circle A22 centre (6.35, -6.35) radius 1.651 projected
  circle A23 centre (6.35, -44.45) radius 1.651 projected
  circle A24 centre (6.35, -228.6) radius 1.651 projected
  circle A25 centre (6.35, -304.8) radius 1.651 projected
  circle A26 centre (247.65, -6.35) radius 1.651 projected
  circle A27 centre (243.8627, -228.6) radius 1.651 projected
  circle A28 centre (243.8627, -304.8) radius 1.651 projected
  line L0 (254, -314.325) -> (254, -196.85) projected
  line L1 (254, -196.85) -> (342.9, -196.85) projected
  line L2 (342.9, -114.3) -> (342.9, -196.85) projected
  line L3 (254, -114.3) -> (342.9, -114.3) projected
  line L4 (254, 0) -> (254, -114.3) projected
  line L5 (0, 0) -> (254, 0) projected
  line L6 (0, 0) -> (0, -114.3) projected
  line L7 (0, -114.3) -> (-88.9, -114.3) projected
  line L8 (-88.9, -196.85) -> (-88.9, -114.3) projected
  line L9 (0, -196.85) -> (-88.9, -196.85) projected
  line L10 (0, -363.855) -> (0, -196.85) projected
  line L11 (285.75, -363.855) -> (0, -363.855) projected
  line L12 (285.75, -314.325) -> (285.75, -363.855) projected
  line L13 (254, -314.325) -> (285.75, -314.325) projected
  point P0 (0, -330.2)
  point P1 (42.7228, -162.052)
  point P2 (42.7228, -189.0014)
  dimension "d345" = 42.7228
  dimension "d346" = 42.7228
  dimension "d347" = 26.9494
  dimension "d348" = 162.052
  measures "d345" distance from line of L6 point (42.723, -162.052)
  measures "d346" distance from line of L6 point (42.723, -189.001)
  measures "d347" distance of point (42.723, -189.001) point (42.723, -162.052)
  measures "d348" distance from line of L5 point (42.723, -162.052)
hole "Hole10" at (42.7228, 168.148, 6.35) at (42.7228, 141.1986, 6.35) direction (0, 0, -1) diameter 3.556 depth 25.4 tip angle 118
body "Solid1"
